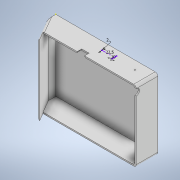
# Autodesk Inventor part: Case
Saved by Autodesk Inventor 2021 (Build 250183000, 183)
## iProperties
Created: 2020-08-28
Part Number: Case
Material: Generisch
Document SubType Name: Modeling
Designer: michox
Density: 1 g/cm^3
Appearance: Vorgabe
Author: michox
Autodesk Inventor part; units mm, degrees
ref_plane "YZ Plane" through (0, 0, 0) normal (1, 0, 0) x (0, 1, 0)
ref_plane "XZ Plane" through (0, 0, 0) normal (0, 1, 0) x (-1, 0, 0)
ref_plane "XY Plane" through (0, 0, 0) normal (0, 0, 1) x (1, 0, 0)
sketch "Skizze1" plane through (0, 0, 0) normal (0, 0, 1) x (1, 0, 0)
  line L0 (0, 0) -> (190.176, 0)
  line L1 (190.176, 0) -> (190.176, -132.329)
  line L2 (190.176, -132.329) -> (0, -132.329)
  line L3 (0, -132.329) -> (0, 0)
  dimension "d0" = 190.176
  dimension "d1" = 132.329
  constraints: 8 end point, 2 parallel, 1 horizontal, 1 perpendicular
  measures "d0" distance of L1.end L2.end
  measures "d1" distance of L0.end L1.end
extrude "Extrusion1" add sketch "Skizze1" along normal blind 55
chamfer "Fase1" distance 38 angle 30 1 edges at (0, -66.1645, 55) measured on face at (0, -66.1645, 54.5)
shell "Wandung1" thickness 2.5 removed faces 1 at (78.0182, -44.1097, 55)
sketch "Skizze2" plane through (0, 0, 55) normal (0, 0, 1) x (1, 0, 0)
  line L0 (24.8261, -129.829) -> (24.8261, -2.5) projected
  line L1 (24.8261, -2.5) -> (24.8261, 0)
  line L2 (24.8261, 0) -> (24.8261, -129.829)
  line L3 (24.8261, -129.829) -> (24.8261, -188.5143)
  line L4 (24.8209, -128.0378) -> (24.8209, -2.5)
  line L5 (24.8209, -2.5) -> (132.5, -2.5)
  line L6 (132.5, -2.5) -> (132.5, -128.0378)
  line L7 (132.5, -128.0378) -> (24.8209, -128.0378)
  line L8 (21.9639, -188.5143) -> (21.9639, 0)
  line L9 (21.9639, -188.5143) -> (24.8261, -188.5143)
  line L10 (197.2096, -151.7277) -> (197.2096, 0)
  line L11 (197.2096, 0) -> (24.8261, 0)
  line L12 (24.8261, -188.5143) -> (197.2096, -151.7277)
  line L13 (24.8261, 0) -> (21.9639, 0)
  point P0 (0, 0)
  point P1 (24.8261, -2.5)
  point P2 (24.8261, -129.8427)
  constraints: 26 end point, 1 collinear, 1 point on line, 1 vertical
extrude "Extrusion2" cut sketch "Skizze2" against normal blind 15 contours L0 L7 L6 L5 L1 L11 L10 L12 L3
sketch "Skizze4" plane through (187.676, -129.829, 2.5) normal (-1, 0, 0) x (0, 0, 1)
  line L0 (31.5, 106.2233) -> (35, 106.2233)
  line L1 (35, 106.2233) -> (35, 21.1057)
  line L2 (35, 21.1057) -> (31.5, 21.1057)
  line L3 (31.5, 21.1057) -> (31.5, 106.2233)
  line L4 (0, 0) -> (0, 127.329) projected
  line L5 (0, 63.6645) -> (37.5, 63.6645)
  line L6 (37.5, 0) -> (37.5, 127.329) projected
  line L7 (37.5, 129.829) -> (37.5, -2.5) projected
  point P0 (-2.5, 129.829)
  point P1 (37.5, 59.7124)
  dimension "d22" = 2.5
  dimension "d51" = 3.5
  constraints: 10 end point, 2 midpoint, 2 parallel, 1 horizontal, 1 perpendicular, 1 other
  measures "d22" distance between parallel lines of L1 L7
  measures "d51" distance of L0.start L0.end
extrude "Extrusion3" cut sketch "Skizze4" against normal blind 1
sketch "Skizze5" plane through (0, -132.329, 0) normal (0, -1, 0) x (1, 0, 0)
  line L0 (187.676, 40) -> (24.8261, 40) projected
  line L1 (24.9479, 55.211) -> (24.9479, 55.211)
  line L2 (2.5, 16.3301) -> (24.8261, 55) projected
  line L3 (24.8261, 40) -> (187.676, 40) projected
  line L4 (24.8261, 40) -> (16.1658, 40)
  line L5 (24.8261, 55) -> (2.5, 16.3301) projected
  line L6 (24.8261, 55) -> (24.8261, 40)
  point P0 (0, 0)
  point P1 (19.3412, 37.9667)
  point P2 (135.0429, 40)
  point P3 (3.1754, 2.5)
  constraints: 6 end point, 1 perpendicular, 1 point on line, 3 other
extrude "Extrusion4" cut sketch "Skizze5" against normal through all
sketch "Skizze7" plane through (0, 0, 0) normal (0, 0, -1) x (-1, 0, 0)
  line L0 (0, -74.1645) -> (6.5147, -74.1645)
  line L1 (14.5147, -66.1645) -> (14.5147, -66.1645)
  line L2 (6.5147, -58.1645) -> (0, -58.1645)
  line L3 (0, -58.1645) -> (0, -74.1645)
  line L4 (-21.9393, -132.329) -> (-21.9393, 0) projected
  line L5 (-21.9393, -66.1645) -> (18.5624, -66.1645)
  circle A0 centre (6.5147, -66.1645) radius 3
  arc A1 (6.5147, -74.1645) -> (14.5147, -66.1645) centre (6.5147, -66.1645) ccw
  arc A2 (14.5147, -66.1645) -> (6.5147, -58.1645) centre (6.5147, -66.1645) ccw
  point P0 (0, 0)
  point P1 (0, -66.1645)
  point P2 (3.5147, -66.1645)
  point P3 (9.5147, -66.1645)
  point P4 (12.5147, -35)
  dimension "d28" = 6
  dimension "d29" = 8
  dimension "d30" = 8
  dimension "d31" = 8
  constraints: 10 end point, 4 point on circle, 4 tangent, 3 centre point, 2 horizontal, 2 parallel, 1 concentric, 1 midpoint, 1 perpendicular, 1 point on line, 1 other
  measures "d28" diameter of A0
  measures "d29" radius of A1
  measures "d30" distance from line of L0 A0.centre
  measures "d31" distance from line of L1 A0.centre
extrude "Extrusion6" add sketch "Skizze7" against normal blind 4 contours L3 L5 A0 A1 L0 | L3 L2 A2 L5 A0
fillet "Rundung1" radius 4.75 2 edges at (0, -58.1645, 2) (0, -74.1645, 2)
fillet "Rundung2" radius 4.75 7 edges at (21.9393, -66.1645, 55) (10.9697, -132.329, 36) (10.9697, 0, 36) (190.176, 0, 20) (190.176, -132.329, 20) (187.676, -129.829, 21.25) (187.676, -2.5, 21.25)
sketch "Skizze9" plane through (0, 0, 0) normal (0, -1, 0) x (1, 0, 0)
  circle A0 centre (100.6662, 14.858) radius 1
  line L0 (124.1662, 9.858) -> (123.1662, 9.858)
  line L1 (123.1662, 9.858) -> (123.1662, 19.858)
  line L2 (123.1662, 19.858) -> (124.1662, 19.858)
  line L3 (124.1662, 19.858) -> (124.1662, 9.858)
  line L4 (100.6662, 14.858) -> (116.0268, 14.858)
  point P0 (0, 0)
  dimension "d43" = 1
  dimension "d44" = 10
  dimension "d45" = 22.5
  dimension "d52" = 2
  constraints: 10 end point, 2 horizontal, 2 parallel, 1 centre point, 1 perpendicular, 1 other
  measures "d43" distance of L1.end L2.end
  measures "d44" distance of L0.end L1.end
  measures "d45" distance from line of L4.start L1
  measures "d52" diameter of A0
extrude "Extrusion7" [suppressed]
sketch "Skizze10" plane through (190.176, -127.579, 0) normal (1, 0, 0) x (0, 0, -1)
  line L0 (-40, 2.5) -> (-40, 120.329) projected
  arc A0 (-40, 110.8457) -> (-40, 122.8457) centre (-39.9533, 116.8457) ccw
  line L1 (-40, 110.8457) -> (-40, 122.8457)
  point P0 (0, 127.579)
  dimension "d48" = 12
  constraints: 2 end point, 2 point on circle, 1 centre point, 1 point on line, 1 vertical
  measures "d48" distance of L1.end L1.start
extrude "Extrusion8" cut sketch "Skizze10" against normal blind 10
sketch "Skizze11" plane through (0, 0, 0) normal (0, 1, 0) x (1, 0, 0)
  line L0 (185.426, 0) -> (185.426, -40) projected
  point P0 (0, 0)
  point P1 (163.426, -15.9242)
  dimension "d60" = 22
  measures "d60" distance from line of L0 point (163.426, -15.924)
hole "Bohrung3" at (163.426, 0, 15.9242) direction (0, -1, 0) diameter 2 depth 5
sketch "Skizze12" plane through (0, 0, 0) normal (0, 1, 0) x (1, 0, 0)
  line L0 (185.426, -40) -> (18.7639, -40) projected
  line L1 (80, -40) -> (93.8, -40)
  line L2 (93.8, -40) -> (93.8, -31.5)
  line L3 (93.8, -31.5) -> (80, -31.5)
  line L4 (80, -31.5) -> (80, -40)
  line L5 (0, 0) -> (0, -7.5) projected
  point P0 (93.8, -40)
  dimension "d61" = 13.8
  dimension "d62" = 8.5
  dimension "d71" = 80
  constraints: 8 end point, 2 parallel, 1 horizontal, 1 perpendicular, 1 point on line
  measures "d61" distance of L3.end L2.end
  measures "d62" distance of L1.end L2.end
  measures "d71" distance between parallel lines of L4 L5
extrude "Extrusion9" cut sketch "Skizze12" against normal blind 10
chamfer "Fase2" distance 2 angle 30 1 edges at (80, -2.5, 35.75) measured on face at (80, -2, 35.75)
chamfer "Fase3" distance 2 angle 30 1 edges at (93.8, -2.5, 35.75) measured on face at (93.8, -2, 35.75)
